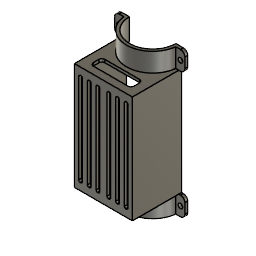
Esc_bracket (Autodesk Fusion 360 design; units mm, degrees)
Autodesk Fusion 360 part; units mm, degrees
sketch "Sketch1" plane through (0, 0, 0) normal (0, 0, 1) x (1, 0, 0)
  circle A0 centre (0, 0) radius 15
  line L0 (-15, 0) -> (15, 0)
  line L1 (15, 0) -> (15, 32)
  line L2 (-15, 32) -> (-15, 0)
  line L3 (-15, 0) -> (15, 0)
  line L4 (15, 0) -> (15, -32)
  line L5 (-15, -32) -> (-15, 0)
  line L6 (-15, -5) -> (-14.1421, -5)
  line L7 (14.1421, -5) -> (15, -5)
  line L8 (-15, 5) -> (-14.1421, 5)
  line L9 (14.1421, 5) -> (15, 5)
  line L10 (-20, 34) -> (-20, -34)
  line L11 (20, 34) -> (20, -34)
  line L12 (-20, 34) -> (20, 34)
  line L13 (-20, -34) -> (20, -34)
  line L14 (18, 32) -> (18, -32)
  line L15 (-18, -32) -> (18, -32)
  line L16 (-18, 32) -> (-18, -32)
  line L17 (-18, 32) -> (18, 32)
  dimension "d1" = 30
  dimension "d9" = 40
  dimension "d10" = 40
  dimension "d11" = 68
  dimension "d12" = -2
  constraint coincident A0.centre origin
  constraint horizontal L0
  constraint vertical L1
  constraint vertical L2
  constraint coincident A0 L0.start
  constraint horizontal L3
  constraint vertical L4
  constraint vertical L5
  constraint coincident A0 L6.end
  constraint coincident A0 L7.start
  constraint collinear L6 L7
  constraint coincident A0 L8.end
  constraint coincident A0 L9.start
  constraint collinear L8 L9
  constraint coincident L4 L7.end
  constraint coincident L1 L9.end
  constraint coincident L5 L6.start
  constraint coincident L2 L8.start
  constraint perpendicular L11 L12
  constraint perpendicular L11 L13
  constraint coincident L17 L2.start
  constraint coincident L17 L1.end
  constraint coincident L15 L5.start
  constraint coincident L15 L4.end
  measures "d1" diameter of A0
  measures "d9" distance of L10.start L11.start
  measures "d10" distance of L10.end L11.end
  measures "d11" distance of L11.end L11.start
extrude "Extrude1" add sketch "Sketch1" along normal blind 100 contours A0 L0 L3 | A0 L0 L3 makes body 1
extrude "Extrude2" add sketch "Sketch1" along normal blind 35 separate body makes body 2
sketch "Sketch2" plane through (0, 0, 35) normal (0, 0, 1) x (-1, 0, 0)
  line L0 (-18, 32) -> (18, 32)
  line L1 (18, 32) -> (18, -32)
  line L2 (18, -32) -> (-18, -32)
  line L3 (-18, -32) -> (-18, 32)
  line L4 (20, -34) -> (20, 34)
  line L5 (20, 34) -> (-20, 34)
  line L6 (-20, 34) -> (-20, -34)
  line L7 (-20, -34) -> (20, -34)
  line L8 (20, -34) -> (-20, -34)
  line L9 (-20, -34) -> (-20, 34)
  line L10 (-20, 34) -> (20, 34)
  line L11 (20, 34) -> (20, -34)
  circle A0 centre (0, 0) radius 15
  circle A1 centre (0, 0) radius 16
  circle A2 centre (0, 0) radius 18
  line L12 (-12, 21) -> (12, 21)
  line L13 (14, 23) -> (14, 27)
  line L14 (12, 29) -> (-12, 29)
  line L15 (-14, 27) -> (-14, 23)
  line L16 (-14, 21) -> (14, 29) construction
  line L17 (14, 21) -> (-14, 29) construction
  arc A3 (12, 21) -> (14, 23) centre (12, 23) ccw
  arc A4 (14, 27) -> (12, 29) centre (12, 27) ccw
  arc A5 (-14, 23) -> (-12, 21) centre (-12, 23) ccw
  arc A6 (-12, 29) -> (-14, 27) centre (-12, 27) ccw
  point P0 (0, 25)
  dimension "d15" = 30
  dimension "d16" = 1
  dimension "d17" = 2
  dimension "d22" = 2
  constraint horizontal L8
  constraint vertical L9
  constraint horizontal L10
  constraint vertical L11
  constraint coincident L5.end L6.start
  constraint coincident L4.start L7.end
  constraint coincident A0.centre A1.centre
  constraint horizontal L12
  constraint perpendicular L12 L13
  constraint parallel L12 L14
  constraint parallel L13 L15
  constraint coincident L16 P0
  constraint coincident L17 P0
  constraint coincident L17.start L13
  constraint coincident L17.start L12
  constraint tangent L13 A3
  constraint tangent L12 A3
  constraint coincident L16.end L13
  constraint coincident L16.end L14
  constraint tangent L13 A4
  constraint tangent L14 A4
  constraint equal A3 A4
  constraint coincident L16.start L12
  constraint coincident L16.start L15
  constraint tangent L12 A5
  constraint tangent L15 A5
  constraint equal A3 A5
  constraint coincident L17.end L15
  constraint coincident L17.end L14
  constraint tangent L15 A6
  constraint tangent L14 A6
  constraint equal A3 A6
  measures "d15" diameter of A0
  measures "d22" radius of A3
extrude "Extrude3" add sketch "Sketch2" along normal blind 2 contours L0 L1 L3 A2 | L1 L2 L3 A2 | L4 L5 L6 L7 L8 L9 L10 L11 | L12 L13 L14 L15 A3 A4 A5 A6 bodies 2
extrude "Extrude4" add sketch "Sketch2" along normal blind 15 contours A2 bodies 2
extrude "Extrude5" cut sketch "Sketch2" along normal blind 2 contours L12 L13 L14 L15 A3 A4 A5 A6 bodies 2
mirror "Mirror1" about plane through (0, 0, 0) normal (0, 1, 0) of "Extrude5"
mirror "Mirror2" about plane through (0, 0, 0) normal (0, 0, 1) of bodies 2 merged
sketch "Sketch3" plane through (0, -34, 0) normal (0, -1, 0) x (1, 0, 0)
  line L0 (20, -37) -> (20, 37)
  line L1 (20, 37) -> (-20, 37)
  line L2 (-20, 37) -> (-20, -37)
  line L3 (-20, -37) -> (20, -37)
  line L4 (0, 0) -> (0, 32.3113)
  line L5 (3.5, 32) -> (4, 32)
  line L6 (5, 31) -> (5, -31)
  line L7 (4, -32) -> (3.5, -32)
  line L8 (2.5, -31) -> (2.5, 31)
  line L9 (-20, 37) -> (20, 37)
  line L10 (20, 37) -> (20, -37)
  line L11 (20, -37) -> (-20, -37)
  line L12 (-20, -37) -> (-20, 37)
  arc A0 (3.5, 32) -> (2.5, 31) centre (3.5, 31) ccw
  arc A1 (5, 31) -> (4, 32) centre (4, 31) ccw
  arc A2 (2.5, -31) -> (3.5, -32) centre (3.5, -31) ccw
  arc A3 (4, -32) -> (5, -31) centre (4, -31) ccw
  line L13 (10, -32) -> (9.5, -32)
  line L14 (11, 31) -> (11, -31)
  line L15 (8.5, -31) -> (8.5, 31)
  arc A4 (11, 31) -> (10, 32) centre (10, 31) ccw
  line L16 (9.5, 32) -> (10, 32)
  arc A5 (10, -32) -> (11, -31) centre (10, -31) ccw
  arc A6 (8.5, -31) -> (9.5, -32) centre (9.5, -31) ccw
  arc A7 (9.5, 32) -> (8.5, 31) centre (9.5, 31) ccw
  line L17 (16, -32) -> (15.5, -32)
  line L18 (17, 31) -> (17, -31)
  line L19 (14.5, -31) -> (14.5, 31)
  arc A8 (17, 31) -> (16, 32) centre (16, 31) ccw
  line L20 (15.5, 32) -> (16, 32)
  arc A9 (16, -32) -> (17, -31) centre (16, -31) ccw
  arc A10 (14.5, -31) -> (15.5, -32) centre (15.5, -31) ccw
  arc A11 (15.5, 32) -> (14.5, 31) centre (15.5, 31) ccw
  line L21 (-4, -32) -> (-3.5, -32)
  line L22 (-17, 31) -> (-17, -31)
  line L23 (-11, 31) -> (-11, -31)
  line L24 (-14.5, -31) -> (-14.5, 31)
  line L25 (-8.5, -31) -> (-8.5, 31)
  arc A12 (-15.5, -32) -> (-14.5, -31) centre (-15.5, -31) ccw
  arc A13 (-14.5, 31) -> (-15.5, 32) centre (-15.5, 31) ccw
  line L26 (-9.5, 32) -> (-10, 32)
  line L27 (-15.5, 32) -> (-16, 32)
  arc A14 (-2.5, 31) -> (-3.5, 32) centre (-3.5, 31) ccw
  line L28 (-3.5, 32) -> (-4, 32)
  arc A15 (-8.5, 31) -> (-9.5, 32) centre (-9.5, 31) ccw
  arc A16 (-10, 32) -> (-11, 31) centre (-10, 31) ccw
  arc A17 (-3.5, -32) -> (-2.5, -31) centre (-3.5, -31) ccw
  arc A18 (-4, 32) -> (-5, 31) centre (-4, 31) ccw
  arc A19 (-17, -31) -> (-16, -32) centre (-16, -31) ccw
  line L29 (-5, 31) -> (-5, -31)
  line L30 (-16, -32) -> (-15.5, -32)
  arc A20 (-11, -31) -> (-10, -32) centre (-10, -31) ccw
  line L31 (-10, -32) -> (-9.5, -32)
  arc A21 (-5, -31) -> (-4, -32) centre (-4, -31) ccw
  arc A22 (-9.5, -32) -> (-8.5, -31) centre (-9.5, -31) ccw
  line L32 (-2.5, -31) -> (-2.5, 31)
  arc A23 (-16, 32) -> (-17, 31) centre (-16, 31) ccw
  dimension "d29" = 5
  dimension "d30" = 5
  dimension "d31" = 1
  dimension "d32" = 1
  dimension "d33" = 1
  constraint coincident L4.start origin
  constraint parallel L2 L4
  constraint horizontal L5
  constraint vertical L6
  constraint horizontal L7
  constraint vertical L8
  constraint horizontal L9
  constraint vertical L10
  constraint horizontal L11
  constraint vertical L12
  constraint coincident L0.start L3.end
  constraint coincident L1.end L2.start
  constraint tangent L8 A0
  constraint tangent L5 A0
  constraint tangent L6 A1
  constraint tangent L5 A1
  constraint equal A0 A1
  constraint tangent L7 A2
  constraint tangent L8 A2
  constraint equal A0 A2
  constraint tangent L6 A3
  constraint tangent L7 A3
  constraint equal A0 A3
  constraint horizontal L16
  constraint vertical L14
  constraint horizontal L13
  constraint vertical L15
  constraint tangent L15 A7
  constraint tangent L16 A7
  constraint tangent L14 A4
  constraint tangent A4 L16
  constraint equal A4 A7
  constraint tangent L13 A6
  constraint tangent L15 A6
  constraint equal A6 A7
  constraint tangent L14 A5
  constraint tangent L13 A5
  constraint equal A5 A7
  constraint horizontal L20
  constraint vertical L18
  constraint horizontal L17
  constraint vertical L19
  constraint tangent L19 A11
  constraint tangent L20 A11
  constraint tangent L18 A8
  constraint tangent A8 L20
  constraint equal A8 A11
  constraint tangent L17 A10
  constraint tangent L19 A10
  constraint equal A10 A11
  constraint tangent L18 A9
  constraint tangent L17 A9
  constraint equal A9 A11
  constraint symmetric L4 L8.end A14.start
  constraint symmetric L4 L5.start A14.end
  constraint symmetric L4 A0 A14
  constraint symmetric L4 L6.start A18.end
  constraint symmetric L4 L5.end L28.end
  constraint symmetric L4 A1 A18
  constraint symmetric L4 L7.end L21.end
  constraint symmetric L4 L8.start A17.end
  constraint symmetric L4 A2 A17
  constraint symmetric L4 L6.end L29.end
  constraint symmetric L4 L7.start L21.start
  constraint symmetric L4 A3 A21
  constraint symmetric L4 L15.end L25.end
  constraint symmetric L4 L16.start L26.start
  constraint symmetric L4 L13.end L31.end
  constraint symmetric L4 A4.end L26.end
  constraint symmetric L4 L14.start L23.start
  constraint symmetric L4 L15.start L25.start
  constraint symmetric L4 L13.start A20.end
  constraint symmetric L4 L14.end L23.end
  constraint symmetric L4 A4 A16
  constraint symmetric L4 A5 A20
  constraint symmetric L4 A6 A22
  constraint symmetric L4 A7 A15
  constraint symmetric L4 L19.end L24.end
  constraint symmetric L4 L20.start A13.end
  constraint symmetric L4 L17.end A12.start
  constraint symmetric L4 A8.end L27.end
  constraint symmetric L4 L18.start L22.start
  constraint symmetric L4 L19.start L24.start
  constraint symmetric L4 L17.start A19.end
  constraint symmetric L4 L18.end L22.end
  constraint symmetric L4 A8 A23
  constraint symmetric L4 A9 A19
  constraint symmetric L4 A10 A12
  constraint symmetric L4 A11 A13
  measures "d29" distance of L5 L9
  measures "d30" distance of L7 L11
  measures "d31" radius of A0
  measures "d32" radius of A7
  measures "d33" radius of A11
extrude "Extrude6" cut sketch "Sketch3" against normal blind 70 contours L5 L6 L7 L8 A0 A1 A2 A3 | L13 L14 L15 A4 L16 A5 A6 A7 | L17 L18 L19 A8 L20 A9 A10 A11 | L21 A14 L28 A17 A18 L29 A21 L32 | L22 L24 A12 A13 L27 A19 L30 A23 | L23 L25 L26 A15 A16 A20 L31 A22 bodies 2
extrude "Extrude7" add 1 faces at (3.0326, -3.9753, 0) along direction (0, 0, -1) blind 80 on bodies 1 bodies 1
split "Split1" by plane through (0, 0, 0) normal (0, 1, 0) bodies 2 makes body 3 at (-20, 22.6667, -12.3333)
sketch "Sketch4" plane through (0, 0, 0) normal (0, 1, 0) x (1, 0, 0)
  line L0 (18, -37) -> (21.2389, -37)
  line L1 (24.2389, -40) -> (24.2389, -47)
  line L2 (21.2389, -50) -> (18, -50)
  line L3 (18, -50) -> (18, -37)
  arc A0 (24.2389, -40) -> (21.2389, -37) centre (21.2389, -40) ccw
  arc A1 (21.2389, -50) -> (24.2389, -47) centre (21.2389, -47) ccw
  circle A2 centre (21.1195, -43.5) radius 1.6
  line L4 (0, -50) -> (0, -37)
  line L5 (-24.2389, -40) -> (-24.2389, -47)
  line L6 (-18, -37) -> (-21.2389, -37)
  line L7 (-18, -50) -> (-18, -37)
  arc A3 (-24.2389, -47) -> (-21.2389, -50) centre (-21.2389, -47) ccw
  circle A4 centre (-21.1195, -43.5) radius 1.6
  line L8 (-21.2389, -50) -> (-18, -50)
  arc A5 (-21.2389, -37) -> (-24.2389, -40) centre (-21.2389, -40) ccw
  point P0 (21.1195, -43.5)
  point P1 (-21.1195, -43.5)
  dimension "d38" = 3
  dimension "d40" = 3.2
  constraint horizontal L0
  constraint vertical L1
  constraint horizontal L2
  constraint vertical L3
  constraint tangent L1 A0
  constraint tangent L0 A0
  constraint tangent L1 A1
  constraint tangent L2 A1
  constraint equal A0 A1
  constraint coincident P0 A2.centre
  constraint vertical L4
  constraint symmetric L0.start L4 L6.start
  constraint symmetric L2.end L4 L7.start
  constraint symmetric L1.start L4 L5.start
  constraint symmetric L0.end L4 L6.end
  constraint symmetric A0 L4 A5
  constraint symmetric L1.end L4 L5.end
  constraint symmetric L2.start L4 A3.end
  constraint symmetric A1 L4 A3
  constraint symmetric A2 L4 A4
  constraint symmetric P0 L4 P1
  measures "d38" radius of A0
  measures "d40" diameter of A2
extrude "Extrude8" add sketch "Sketch4" along normal blind 2 bodies 3
extrude "Extrude9" add sketch "Sketch4" against normal blind 2 bodies 2
extrude "Extrude10" add 1 faces at (18, 1.3333, 45.6667) along direction (-1, 0, 0) blind 1 on bodies 3 bodies 3
extrude "Extrude11" add 1 faces at (-18, 1.3333, 45.6667) along direction (1, 0, 0) blind 0.1 on bodies 3 bodies 3
split "Split2" by plane through (0, 0, 0) normal (0, 0, 1) bodies 3 makes body 4 at (-20, 12, 12.3333)
delete_body "RemoveBody1" bodies 3
mirror "Mirror3" about plane through (0, 0, 0) normal (0, 0, 1) of bodies 4 merged
delete_body "RemoveBody2" bodies 2
mirror "Mirror4" about plane through (0, 0, 0) normal (0, 1, 0) of bodies 4 makes body 5
hidden bodies 1 4
